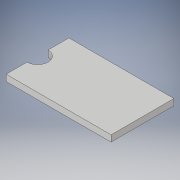
# Autodesk Inventor part: stamp5x3
Saved by Autodesk Inventor 2019 (Build 230136000, 136)
## iProperties
Created: 2019-02-19
Part Number: stamp5x3
Material: Generic
Document SubType Name: Modeling
Designer: jmc
Density: 1 g/cm^3
Appearance: Default
Author: jmc
Autodesk Inventor part; units mm, degrees
ref_plane "YZ Plane" through (0, 0, 0) normal (1, 0, 0) x (0, 1, 0)
ref_plane "XZ Plane" through (0, 0, 0) normal (0, 1, 0) x (-1, 0, 0)
ref_plane "XY Plane" through (0, 0, 0) normal (0, 0, 1) x (1, 0, 0)
sketch "Sketch1" plane through (0, 0, 0) normal (0, 1, 0) x (-1, 0, 0)
  line L0 (24.925, 14.925) -> (-24.925, 14.925)
  line L1 (-24.925, 14.925) -> (-24.925, -14.925)
  line L2 (-24.925, -14.925) -> (24.925, -14.925)
  line L3 (24.925, 14.925) -> (-24.925, -14.925) construction
  line L4 (-24.925, 14.925) -> (24.925, -14.925) construction
  arc A0 (24.925, 5) -> (24.925, -5) centre (24.925, 0) ccw
  line L5 (24.925, -14.925) -> (24.925, -5)
  line L6 (24.925, 5) -> (24.925, 14.925)
  point P0 (0, 0)
  dimension "d0" = 49.85
  dimension "d1" = 29.85
  dimension "d4" = 10
  constraints: 14 end point, 3 parallel, 2 midpoint, 2 point on circle, 1 centre point, 1 horizontal, 1 perpendicular
  measures "d0" distance of L2.end L1.end
  measures "d1" distance of L1.end L0.end
  measures "d4" diameter of A0
extrude "Extrusion1" add sketch "Sketch1" along normal blind 3
body "Solid1"
